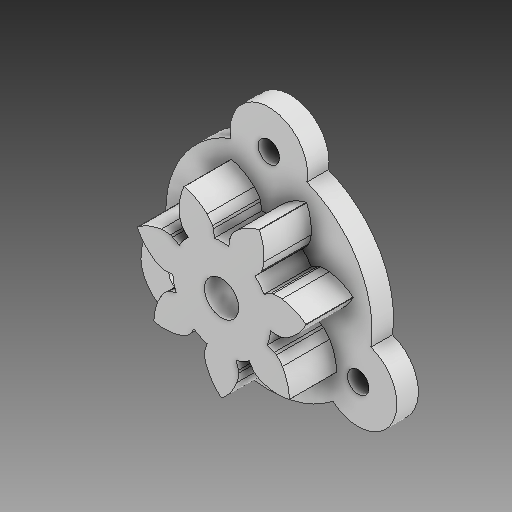
# Autodesk Inventor part: 歯車m2.z7(z19)
Saved by Autodesk Inventor 2020 (Build 240168000, 168)
## iProperties
Created: 2019-09-03
Part Number: 歯車m2.z7(z19)
Material: アルミニウム 2014-T4
Document SubType Name: Modeling
Designer: 雪村
Density: 2.8 g/cm^3
Appearance: サテン
Mass: 6.46025 g
Surface Area: 19.2839 cm^2
Volume: 2.30723 cm^3
Description: アルミ2000 8t
Author: 雪村
Autodesk Inventor part; units mm, degrees
ref_plane "YZ Plane" through (0, 0, 0) normal (1, 0, 0) x (0, 1, 0)
ref_plane "XZ Plane" through (0, 0, 0) normal (0, 1, 0) x (-1, 0, 0)
ref_plane "XY Plane" through (0, 0, 0) normal (0, 0, 1) x (1, 0, 0)
sketch "スケッチ1" plane through (0, 0, 0) normal (0, 0, 1) x (1, 0, 0)
  arc A0 (1.0596, 6.774) -> (0.9641, 6.5068) centre (2.0212, 6.2798) ccw
  arc A1 (1.6991, 7.6367) -> (1.0596, 6.774) centre (3.8299, 5.389) ccw
  arc A2 (4.3402, 9.0752) -> (1.6991, 7.6367) centre (5.7463, 3.3497) ccw
  arc A3 (-4.6355, 5.052) -> (-4.4861, 4.8107) centre (-3.6495, 5.4956) ccw
  arc A4 (-4.9113, 6.0898) -> (-4.6355, 5.052) centre (-1.8254, 6.3543) ccw
  arc A5 (-4.3892, 9.0516) -> (-4.9113, 6.0898) centre (0.9639, 6.5812) ccw
  arc A6 (-6.84, -0.4743) -> (-6.5582, -0.508) centre (-6.5721, 0.5731) ccw
  arc A7 (-7.8233, -0.0429) -> (-6.84, -0.4743) centre (-6.1061, 2.5347) ccw
  arc A8 (-9.8135, 2.2119) -> (-7.8233, -0.0429) centre (-4.5444, 4.8569) ccw
  arc A9 (-3.8938, -5.6435) -> (-3.6918, -5.4441) centre (-4.5457, -4.7809) ccw
  arc A10 (-4.8442, -6.1433) -> (-3.8938, -5.6435) centre (-5.7888, -3.1936) ccw
  arc A11 (-7.848, -6.2934) -> (-4.8442, -6.1433) centre (-6.6307, -0.5248) ccw
  arc A12 (1.9845, -6.5629) -> (1.9546, -6.2807) centre (0.9037, -6.5348) ccw
  arc A13 (1.7827, -7.6176) -> (1.9845, -6.5629) centre (-1.1124, -6.517) ccw
  arc A14 (0.0272, -10.0597) -> (1.7827, -7.6176) centre (-3.7239, -5.5113) ccw
  arc A15 (6.3684, -2.5404) -> (6.1291, -2.3878) centre (5.6726, -3.3679) ccw
  arc A16 (7.0672, -3.3558) -> (6.3684, -2.5404) centre (4.4016, -4.933) ccw
  arc A17 (7.8819, -6.2508) -> (7.0672, -3.3558) centre (1.9871, -6.3477) ccw
  arc A18 (5.9568, 3.3951) -> (5.6883, 3.3032) centre (6.1699, 2.3351) ccw
  arc A19 (7.03, 3.433) -> (5.9568, 3.3951) centre (6.6011, 0.3656) ccw
  arc A20 (9.8014, 2.265) -> (7.03, 3.433) centre (6.2017, -2.4041) ccw
  arc A21 (-0.9641, 6.5068) -> (-1.0596, 6.774) centre (-2.0212, 6.2798) ccw
  arc A22 (-1.0596, 6.774) -> (-1.6991, 7.6367) centre (-3.8299, 5.389) ccw
  arc A23 (-1.6991, 7.6367) -> (-4.3402, 9.0752) centre (-5.7463, 3.3497) ccw
  arc A24 (-5.6883, 3.3032) -> (-5.9568, 3.3951) centre (-6.1699, 2.3351) ccw
  arc A25 (-5.9568, 3.3951) -> (-7.03, 3.433) centre (-6.6011, 0.3656) ccw
  arc A26 (-7.03, 3.433) -> (-9.8014, 2.265) centre (-6.2017, -2.4041) ccw
  arc A27 (-6.1291, -2.3878) -> (-6.3684, -2.5404) centre (-5.6726, -3.3679) ccw
  arc A28 (-6.3684, -2.5404) -> (-7.0672, -3.3558) centre (-4.4016, -4.933) ccw
  arc A29 (-7.0672, -3.3558) -> (-7.8819, -6.2508) centre (-1.9871, -6.3477) ccw
  arc A30 (-1.9546, -6.2807) -> (-1.9845, -6.5629) centre (-0.9037, -6.5348) ccw
  arc A31 (-1.9845, -6.5629) -> (-1.7827, -7.6176) centre (1.1124, -6.517) ccw
  arc A32 (-1.7827, -7.6176) -> (-0.0272, -10.0597) centre (3.7239, -5.5113) ccw
  arc A33 (3.6918, -5.4441) -> (3.8938, -5.6435) centre (4.5457, -4.7809) ccw
  arc A34 (3.8938, -5.6435) -> (4.8442, -6.1433) centre (5.7888, -3.1936) ccw
  arc A35 (4.8442, -6.1433) -> (7.848, -6.2934) centre (6.6307, -0.5248) ccw
  arc A36 (6.5582, -0.508) -> (6.84, -0.4743) centre (6.5721, 0.5731) ccw
  arc A37 (6.84, -0.4743) -> (7.8233, -0.0429) centre (6.1061, 2.5347) ccw
  arc A38 (7.8233, -0.0429) -> (9.8135, 2.2119) centre (4.5444, 4.8569) ccw
  arc A39 (4.4861, 4.8107) -> (4.6355, 5.052) centre (3.6495, 5.4956) ccw
  arc A40 (4.6355, 5.052) -> (4.9113, 6.0898) centre (1.8254, 6.3543) ccw
  arc A41 (4.9113, 6.0898) -> (4.3892, 9.0516) centre (-0.9639, 6.5812) ccw
  arc A42 (0.8355, 5.6384) -> (-0.8355, 5.6384) centre (0, 0) ccw
  arc A43 (-3.8874, 4.1687) -> (-4.9292, 2.8623) centre (0, 0) ccw
  arc A44 (-5.683, -0.4402) -> (-5.3112, -2.0692) centre (0, 0) ccw
  arc A45 (-3.1991, -4.7176) -> (-1.6937, -5.4425) centre (0, 0) ccw
  arc A46 (1.6937, -5.4425) -> (3.1991, -4.7176) centre (0, 0) ccw
  arc A47 (5.3112, -2.0692) -> (5.683, -0.4402) centre (0, 0) ccw
  arc A48 (4.9292, 2.8623) -> (3.8874, 4.1687) centre (0, 0) ccw
  arc A49 (-4.3402, 9.0752) -> (-4.3892, 9.0516) centre (0, 0) ccw
  arc A50 (-9.8014, 2.265) -> (-9.8135, 2.2119) centre (0, 0) ccw
  arc A51 (-7.8819, -6.2508) -> (-7.848, -6.2934) centre (0, 0) ccw
  arc A52 (-0.0272, -10.0597) -> (0.0272, -10.0597) centre (0, 0) ccw
  arc A53 (7.848, -6.2934) -> (7.8819, -6.2508) centre (0, 0) ccw
  arc A54 (9.8135, 2.2119) -> (9.8014, 2.265) centre (0, 0) ccw
  arc A55 (4.3892, 9.0516) -> (4.3402, 9.0752) centre (0, 0) ccw
  line L0 (0.8355, 5.6384) -> (0.9641, 6.5068)
  line L1 (-3.8874, 4.1687) -> (-4.4861, 4.8107)
  line L2 (-5.683, -0.4402) -> (-6.5582, -0.508)
  line L3 (-3.1991, -4.7176) -> (-3.6918, -5.4441)
  line L4 (1.6937, -5.4425) -> (1.9546, -6.2807)
  line L5 (5.3112, -2.0692) -> (6.1291, -2.3878)
  line L6 (4.9292, 2.8623) -> (5.6883, 3.3032)
  line L7 (-0.8355, 5.6384) -> (-0.9641, 6.5068)
  line L8 (-4.9292, 2.8623) -> (-5.6883, 3.3032)
  line L9 (-5.3112, -2.0692) -> (-6.1291, -2.3878)
  line L10 (-1.6937, -5.4425) -> (-1.9546, -6.2807)
  line L11 (3.1991, -4.7176) -> (3.6918, -5.4441)
  line L12 (5.683, -0.4402) -> (6.5582, -0.508)
  line L13 (3.8874, 4.1687) -> (4.4861, 4.8107)
  line L14 (-12.0597, 0) -> (12.0597, 0)
  line L15 (0, -12.0597) -> (0, 12.0597)
  line L16 (30.0597, 10.0597) -> (100.0597, 10.0597)
  line L17 (30.0597, 2.0597) -> (100.0597, 2.0597)
  line L18 (30.0597, -5.9403) -> (100.0597, -5.9403)
  line L19 (30.0597, -13.9403) -> (100.0597, -13.9403)
  line L20 (30.0597, -21.9403) -> (100.0597, -21.9403)
  line L21 (30.0597, -29.9403) -> (100.0597, -29.9403)
  line L22 (30.0597, -37.9403) -> (100.0597, -37.9403)
  line L23 (30.0597, -45.9403) -> (100.0597, -45.9403)
  line L24 (30.0597, -53.9403) -> (100.0597, -53.9403)
  line L25 (30.0597, -61.9403) -> (100.0597, -61.9403)
  line L26 (30.0597, -69.9403) -> (100.0597, -69.9403)
  line L27 (30.0597, -77.9403) -> (100.0597, -77.9403)
  line L28 (30.0597, -85.9403) -> (100.0597, -85.9403)
  line L29 (30.0597, 10.0597) -> (30.0597, -85.9403)
  line L30 (100.0597, 10.0597) -> (100.0597, -85.9403)
  line L31 (65.0597, 2.0597) -> (65.0597, -85.9403)
  point P0 (0, 0)
  point P1 (36.0597, 4.0597)
  point P2 (38.5597, -3.9403)
  point P3 (38.5597, -11.9403)
  point P4 (36.0597, -19.9403)
  point P5 (38.5597, -27.9403)
  point P6 (33.5597, -35.9403)
  point P7 (36.0597, -43.9403)
  point P8 (36.0597, -51.9403)
  point P9 (36.0597, -59.9403)
  point P10 (38.5597, -67.9403)
  point P11 (38.5597, -75.9403)
  point P12 (36.0597, -83.9403)
  point P13 (66.0597, -3.9403)
  point P14 (82.3097, -11.9403)
  point P15 (82.3097, -19.9403)
  point P16 (78.5597, -27.9403)
  point P17 (81.0597, -35.9403)
  point P18 (74.8097, -43.9403)
  point P19 (74.8097, -51.9403)
  point P20 (78.5597, -59.9403)
  point P21 (76.0597, -67.9403)
  point P22 (1, 25.5597)
  point P23 (1, 19.5597)
  point P24 (18.25, 25.5597)
  point P25 (20.375, 19.5597)
  constraints: 112 point on circle, 60 end point, 56 centre point, 14 horizontal, 2 midpoint, 2 vertical, 294 other
extrude "押し出し1" add sketch "スケッチ1" along normal blind 5.5 contours A1 A2 A55 A41 A40 A39 L13 A48 L6 A18 A19 A20 A54 A38 L14 L15 A42 L0 A0 | L15 L14 A8 A50 A26 A25 A24 L8 A43 L1 A3 A4 A5 A49 A23 A22 A21 L7 A42 | L15 A52 A32 A31 A30 L10 A45 L3 A9 A10 A11 A51 A29 A28 A27 L9 A44 L2 A6 A7 A8 L14 | L14 A38 A37 A36 L12 A47 L5 A15 A16 A17 A53 A35 A34 A33 L11 A46 L4 A12 A13 A14 A52 L15
sketch "スケッチ2" plane through (0, 0, 0) normal (0, 0, -1) x (-1, 0, 0)
  circle A0 centre (0, 0) radius 1.995
  line L0 (0, 12) -> (10.3923, -6) construction
  line L1 (10.3923, -6) -> (-10.3923, -6) construction
  line L2 (-10.3923, -6) -> (0, 12) construction
  circle A1 centre (-10.3923, -6) radius 1.25
  circle A2 centre (0, 12) radius 1.25
  circle A3 centre (10.3923, -6) radius 1.25
  arc A4 (-4.3402, 9.0752) -> (-4.3892, 9.0516) centre (0, 0) ccw projected
  circle A5 centre (0, 0) radius 10.0597 construction
  circle A6 centre (0, 0) radius 12
  circle A7 centre (0, 12) radius 4.5
  circle A8 centre (10.3923, -6) radius 4.5
  circle A9 centre (-10.3923, -6) radius 4.5
  circle A10 centre (0, 0) radius 16.5 construction
  point P0 (-11.8717, -1.7501)
  point P1 (-7.4515, -9.4061)
  point P2 (9.7118, -7.0485)
  point P3 (10.9601, -4.8864)
  point P4 (1.2483, 11.9349)
  point P5 (-1.2483, 11.9349)
  point P6 (11.8717, -1.7501)
  point P7 (7.4515, -9.4061)
  point P8 (-4.4202, 11.1563)
  point P9 (4.4202, 11.1563)
  dimension "d2" = 3.99
  dimension "d3" = 2.5
  dimension "d4" = 2.5
  dimension "d5" = 2.5
  dimension "d6" = 12
  dimension "d14" = 9
  dimension "d15" = 9
  dimension "d16" = 9
  constraints: 8 centre point, 8 coincident, 6 end point, 1 horizontal, 1 tangent, 13 other
  measures "d2" diameter of A0
  measures "d3" diameter of A1
  measures "d4" diameter of A2
  measures "d5" diameter of A3
  measures "d6" distance of L0.start A4.centre
  measures "d14" diameter of A9
  measures "d15" diameter of A7
  measures "d16" diameter of A8
extrude "押し出し2" add sketch "スケッチ2" along normal blind 2.5 contours A1 A6 A9 | A1 A6 A9 | A6 A7 A8 A9 | A7 A6 A2 | A6 A2 A7 | A8 A6 A3 | A6 A3 A8
sketch "スケッチ3" plane through (0, 0, 0) normal (0, 0, -1) x (-1, 0, 0)
  circle A0 centre (0, 0) radius 1.995 projected
extrude "押し出し3" cut sketch "スケッチ3" against normal through all
sketch "スケッチ4" plane through (0, 0, 5.5) normal (0, 0, 1) x (1, 0, 0)
  arc A0 (11.8717, -1.7501) -> (4.4202, 11.1563) centre (0, 0) ccw projected
  arc A1 (4.4202, 11.1563) -> (-4.4202, 11.1563) centre (0, 12) ccw projected
  arc A2 (-4.4202, 11.1563) -> (-11.8717, -1.7501) centre (0, 0) ccw projected
  arc A3 (-11.8717, -1.7501) -> (-7.4515, -9.4061) centre (-10.3923, -6) ccw projected
  arc A4 (-7.4515, -9.4061) -> (7.4515, -9.4061) centre (0, 0) ccw projected
  arc A5 (7.4515, -9.4061) -> (11.8717, -1.7501) centre (10.3923, -6) ccw projected
  circle A6 centre (0, 12) radius 1.25 projected
  circle A7 centre (10.3923, -6) radius 1.25 projected
  circle A8 centre (-10.3923, -6) radius 1.25 projected
  arc A9 (7.848, -6.2934) -> (7.8819, -6.2508) centre (0, 0) ccw projected
  arc A10 (4.8442, -6.1433) -> (7.848, -6.2934) centre (6.6307, -0.5248) ccw projected
  arc A11 (3.8938, -5.6435) -> (4.8442, -6.1433) centre (5.7888, -3.1936) ccw projected
  arc A12 (3.6918, -5.4441) -> (3.8938, -5.6435) centre (4.5457, -4.7809) ccw projected
  line L0 (3.1991, -4.7176) -> (3.6918, -5.4441) projected
  arc A13 (1.6937, -5.4425) -> (3.1991, -4.7176) centre (0, 0) ccw projected
  line L1 (1.9546, -6.2807) -> (1.6937, -5.4425) projected
  arc A14 (1.9845, -6.5629) -> (1.9546, -6.2807) centre (0.9037, -6.5348) ccw projected
  arc A15 (1.7827, -7.6176) -> (1.9845, -6.5629) centre (-1.1124, -6.517) ccw projected
  arc A16 (0.0272, -10.0597) -> (1.7827, -7.6176) centre (-3.7239, -5.5113) ccw projected
  arc A17 (-0.0272, -10.0597) -> (0.0272, -10.0597) centre (0, 0) ccw projected
  arc A18 (-1.7827, -7.6176) -> (-0.0272, -10.0597) centre (3.7239, -5.5113) ccw projected
  arc A19 (-1.9845, -6.5629) -> (-1.7827, -7.6176) centre (1.1124, -6.517) ccw projected
  arc A20 (-1.9546, -6.2807) -> (-1.9845, -6.5629) centre (-0.9037, -6.5348) ccw projected
  line L2 (-1.6937, -5.4425) -> (-1.9546, -6.2807) projected
  arc A21 (-3.1991, -4.7176) -> (-1.6937, -5.4425) centre (0, 0) ccw projected
  line L3 (-3.6918, -5.4441) -> (-3.1991, -4.7176) projected
  arc A22 (-3.8938, -5.6435) -> (-3.6918, -5.4441) centre (-4.5457, -4.7809) ccw projected
  arc A23 (-4.8442, -6.1433) -> (-3.8938, -5.6435) centre (-5.7888, -3.1936) ccw projected
  arc A24 (-7.848, -6.2934) -> (-4.8442, -6.1433) centre (-6.6307, -0.5248) ccw projected
  arc A25 (-7.8819, -6.2508) -> (-7.848, -6.2934) centre (0, 0) ccw projected
  arc A26 (-7.0672, -3.3558) -> (-7.8819, -6.2508) centre (-1.9871, -6.3477) ccw projected
  arc A27 (-6.3684, -2.5404) -> (-7.0672, -3.3558) centre (-4.4016, -4.933) ccw projected
  arc A28 (-6.1291, -2.3878) -> (-6.3684, -2.5404) centre (-5.6726, -3.3679) ccw projected
  line L4 (-5.3112, -2.0692) -> (-6.1291, -2.3878) projected
  arc A29 (-5.683, -0.4402) -> (-5.3112, -2.0692) centre (0, 0) ccw projected
  line L5 (-6.5582, -0.508) -> (-5.683, -0.4402) projected
  arc A30 (-6.84, -0.4743) -> (-6.5582, -0.508) centre (-6.5721, 0.5731) ccw projected
  arc A31 (-7.8233, -0.0429) -> (-6.84, -0.4743) centre (-6.1061, 2.5347) ccw projected
  arc A32 (-9.8135, 2.2119) -> (-7.8233, -0.0429) centre (-4.5444, 4.8569) ccw projected
  arc A33 (-9.8014, 2.265) -> (-9.8135, 2.2119) centre (0, 0) ccw projected
  arc A34 (-7.03, 3.433) -> (-9.8014, 2.265) centre (-6.2017, -2.4041) ccw projected
  arc A35 (-5.9568, 3.3951) -> (-7.03, 3.433) centre (-6.6011, 0.3656) ccw projected
  arc A36 (-5.6883, 3.3032) -> (-5.9568, 3.3951) centre (-6.1699, 2.3351) ccw projected
  line L6 (-4.9292, 2.8623) -> (-5.6883, 3.3032) projected
  arc A37 (-3.8874, 4.1687) -> (-4.9292, 2.8623) centre (0, 0) ccw projected
  line L7 (-4.4861, 4.8107) -> (-3.8874, 4.1687) projected
  arc A38 (-4.6355, 5.052) -> (-4.4861, 4.8107) centre (-3.6495, 5.4956) ccw projected
  arc A39 (-4.9113, 6.0898) -> (-4.6355, 5.052) centre (-1.8254, 6.3543) ccw projected
  arc A40 (-4.3892, 9.0516) -> (-4.9113, 6.0898) centre (0.9639, 6.5812) ccw projected
  arc A41 (-4.3402, 9.0752) -> (-4.3892, 9.0516) centre (0, 0) ccw projected
  arc A42 (-1.6991, 7.6367) -> (-4.3402, 9.0752) centre (-5.7463, 3.3497) ccw projected
  arc A43 (-1.0596, 6.774) -> (-1.6991, 7.6367) centre (-3.8299, 5.389) ccw projected
  arc A44 (-0.9641, 6.5068) -> (-1.0596, 6.774) centre (-2.0212, 6.2798) ccw projected
  line L8 (-0.8355, 5.6384) -> (-0.9641, 6.5068) projected
  arc A45 (0.8355, 5.6384) -> (-0.8355, 5.6384) centre (0, 0) ccw projected
  line L9 (0.9641, 6.5068) -> (0.8355, 5.6384) projected
  arc A46 (1.0596, 6.774) -> (0.9641, 6.5068) centre (2.0212, 6.2798) ccw projected
  arc A47 (1.6991, 7.6367) -> (1.0596, 6.774) centre (3.8299, 5.389) ccw projected
  arc A48 (4.3402, 9.0752) -> (1.6991, 7.6367) centre (5.7463, 3.3497) ccw projected
  arc A49 (4.3892, 9.0516) -> (4.3402, 9.0752) centre (0, 0) ccw projected
  arc A50 (4.9113, 6.0898) -> (4.3892, 9.0516) centre (-0.9639, 6.5812) ccw projected
  arc A51 (4.6355, 5.052) -> (4.9113, 6.0898) centre (1.8254, 6.3543) ccw projected
  arc A52 (4.4861, 4.8107) -> (4.6355, 5.052) centre (3.6495, 5.4956) ccw projected
  line L10 (3.8874, 4.1687) -> (4.4861, 4.8107) projected
  arc A53 (4.9292, 2.8623) -> (3.8874, 4.1687) centre (0, 0) ccw projected
  line L11 (5.6883, 3.3032) -> (4.9292, 2.8623) projected
  arc A54 (5.9568, 3.3951) -> (5.6883, 3.3032) centre (6.1699, 2.3351) ccw projected
  arc A55 (7.03, 3.433) -> (5.9568, 3.3951) centre (6.6011, 0.3656) ccw projected
  arc A56 (9.8014, 2.265) -> (7.03, 3.433) centre (6.2017, -2.4041) ccw projected
  arc A57 (9.8135, 2.2119) -> (9.8014, 2.265) centre (0, 0) ccw projected
  arc A58 (7.8233, -0.0429) -> (9.8135, 2.2119) centre (4.5444, 4.8569) ccw projected
  arc A59 (6.84, -0.4743) -> (7.8233, -0.0429) centre (6.1061, 2.5347) ccw projected
  arc A60 (6.5582, -0.508) -> (6.84, -0.4743) centre (6.5721, 0.5731) ccw projected
  line L12 (5.683, -0.4402) -> (6.5582, -0.508) projected
  arc A61 (5.3112, -2.0692) -> (5.683, -0.4402) centre (0, 0) ccw projected
  line L13 (6.1291, -2.3878) -> (5.3112, -2.0692) projected
  arc A62 (6.3684, -2.5404) -> (6.1291, -2.3878) centre (5.6726, -3.3679) ccw projected
  arc A63 (7.0672, -3.3558) -> (6.3684, -2.5404) centre (4.4016, -4.933) ccw projected
  arc A64 (7.8819, -6.2508) -> (7.0672, -3.3558) centre (1.9871, -6.3477) ccw projected
  circle A65 centre (0, 0) radius 1.995 projected
equation "\"d4\" = d3"
equation "\"d5\" = d4"
